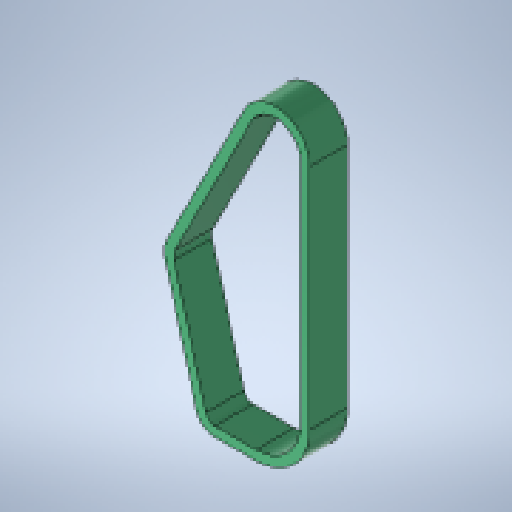
# Autodesk Inventor part: Temp Tread
Saved by Autodesk Inventor 2023.4 (Build 274418000, 418)
## iProperties
Created: 2024-05-07
Part Number: Temp Tread
Material: Rubber, Silicone
Document SubType Name: Modeling
Designer: Nathan Cai
Density: 1.25 g/cm^3
Appearance: Smooth - Dark Sea Green
Author: Nathan Cai
Autodesk Inventor part; units mm, degrees
ref_plane "YZ Plane" through (0, 0, 0) normal (1, 0, 0) x (0, 1, 0)
ref_plane "XZ Plane" through (0, 0, 0) normal (0, 1, 0) x (-1, 0, 0)
ref_plane "XY Plane" through (0, 0, 0) normal (0, 0, 1) x (1, 0, 0)
sketch "Sketch1" plane through (0, 0, 0) normal (0, 0, 1) x (1, 0, 0)
  arc A0 (0, -22.225) -> (22.225, 0) centre (0, 0) ccw
  arc A1 (22.225, 114.3) -> (-1.7838, 120.0793) centre (9.525, 114.3) ccw
  line L0 (22.225, 114.3) -> (22.225, 0)
  arc A2 (-40.5794, 44.1646) -> (-41.0519, 39.6067) centre (-34.925, 41.275) ccw
  line L1 (-1.7838, 120.0793) -> (-40.5794, 44.1646)
  arc A3 (-25.1715, -18.7137) -> (-20.5764, -22.225) centre (-20.5764, -17.4625) ccw
  line L2 (-20.5764, -22.225) -> (0, -22.225)
  line L3 (-41.0519, 39.6067) -> (-25.1715, -18.7137)
  arc A4 (-29.7667, -19.965) -> (-20.5764, -26.9875) centre (-20.5764, -17.4625) ccw
  line L4 (-20.5764, -26.9875) -> (0, -26.9875)
  arc A5 (0, -26.9875) -> (26.9875, 0) centre (0, 0) ccw
  line L5 (26.9875, 0) -> (26.9875, 114.3)
  arc A6 (26.9875, 114.3) -> (-6.0247, 122.2465) centre (9.525, 114.3) ccw
  line L6 (-6.0247, 122.2465) -> (-44.8202, 46.3319)
  arc A7 (-44.8202, 46.3319) -> (-45.6471, 38.3554) centre (-34.925, 41.275) ccw
  line L7 (-45.6471, 38.3554) -> (-29.7667, -19.965)
  dimension "d0" = 44.45
  dimension "d1" = 25.4
  dimension "d2" = 114.3
  dimension "d3" = 12.7
  dimension "d4" = 41.275
  dimension "d5" = 34.925
  dimension "d6" = 9.525
  dimension "d7" = 4.7625
  constraints: 16 end point, 16 point on circle, 9 tangent, 8 centre point, 1 coincident, 1 horizontal, 1 vertical, 7 other
  measures "d0" diameter of A0
  measures "d1" diameter of A1
  measures "d2" vertical distance of point (0, 0) A1.centre
  measures "d3" diameter of A2
  measures "d4" vertical distance of A0.centre A2.centre
  measures "d5" horizontal distance of A0.centre A2.centre
  measures "d6" diameter of A3
  measures "d7" distance between parallel lines of L3 L7
extrude "Extrusion1" add sketch "Sketch1" along normal blind 19.05
body "Solid1"
